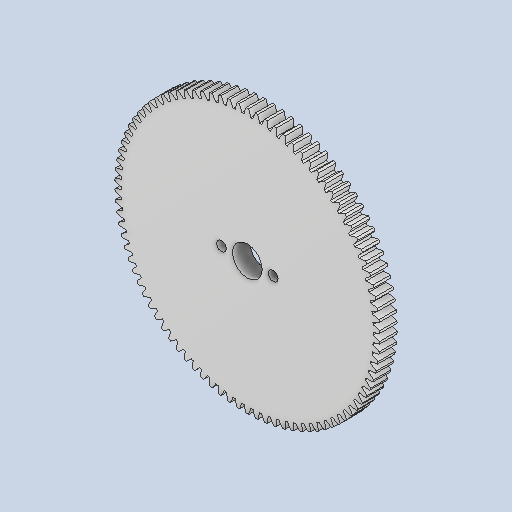
# Autodesk Inventor part: 平歯車1
Saved by Autodesk Inventor 2025.2 (Build 292293000, 293)
## iProperties
CustomPartVersion: 1
Created: 2024-12-08
Part Number: 平歯車1
Material: ABS プラスチック
Document SubType Name: Modeling
Designer: haruy
Categories: <?xml version="1.0" encoding="UTF-16"?> <MemberInstance><Categories><FamilyTemplate><FamilyTemplateParameter ValueType="xs:double" Id="1" ObjectReferenceKey="da_z" ObjectType="kUserParameterObject"/><FamilyTemplateParameter ValueType="xs:double" Id="2" ObjectReferenceKey="da_b" ObjectType="kUserParameterObject"/><FamilyTemplateParameter ValueType="xs:double" Id="3" ObjectReferenceKey="da_beta" ObjectType="kUserParameterObject"/><FamilyTemplateParameter ValueType="xs:double" Id="4" ObjectReferenceKey="da_da" ObjectType="kUserParameterObject"/><FamilyTemplateParameter ValueType="xs:double" Id="5" ObjectReferenceKey="da_aw" ObjectType="kUserParameterObject"/><FamilyTemplateParameter ValueType="xs:string" Id="6" ObjectReferenceKey="EAIAABAAAACIAQAAAAAAAIAAAAAAAAAA" ObjectType="83910656" SubObjectId="SurfaceGeometry"/></FamilyTemplate><ParamToTemplateMap><ParamToTemplate CategoryParameter="//CategoryParameter[@InternalName='046C89C9-8512-4d59-83FE-43B91F4F132A']" TemplateParameter="1"/><ParamToTemplate CategoryParameter="//CategoryParameter[@InternalName='2552DF32-E462-4b46-AEBF-C6C7768E72AC']" TemplateParameter="2"/><ParamToTemplate CategoryParameter="//CategoryParameter[@InternalName='C9EE641D-15FC-4fae-A226-E94C4372FDD7']" TemplateParameter="3"/><ParamToTemplate><ParamToTemplate CategoryParameter="//CategoryParameter[@InternalName='00B6519A-459B-49c7-AD84-2E56D39A5744']" ConstantValue="0.000000"/></ParamToTemplate><ParamToTemplate><ParamToTemplate CategoryParameter="//CategoryParameter[@InternalName='04B31F0E-C7A6-4894-AA32-9629BEFACF47']" ConstantValue="1.000000"/></ParamToTemplate><ParamToTemplate><ParamToTemplate CategoryParameter="//CategoryParameter[@InternalName='43CBEC2E-7847-49e7-A936-2F7889FCB2D9']" ConstantValue="0.250000"/></ParamToTemplate><ParamToTemplate><ParamToTemplate CategoryParameter="//CategoryParameter[@InternalName='B1EFC894-105D-4ebd-86BF-FA20ED196853']" ConstantValue="0.350000"/></ParamToTemplate><ParamToTemplate><ParamToTemplate CategoryParameter="//CategoryParameter[@InternalName='51175063-3D10-4879-93E8-6246FE8B403D']" ConstantValue="2060000000.000000"/></ParamToTemplate><ParamToTemplate><ParamToTemplate CategoryParameter="//CategoryParameter[@InternalName='A3A52E27-4454-46a9-B0BD-C932399B70AF']" ConstantValue="0.300000"/></ParamToTemplate><ParamToTemplate><ParamToTemplate CategoryParameter="//CategoryParameter[@InternalName='91B76062-C214-41d9-B1B9-14D2AB99603D']" ConstantValue="0.100000"/></ParamToTemplate><ParamToTemplate><ParamToTemplate CategoryParameter="//CategoryParameter[@InternalName='374E806E-8B8A-4dda-A9AA-1039D6500AD2']" ConstantValue="10.000000"/></ParamToTemplate><ParamToTemplate><ParamToTemplate CategoryParameter="//CategoryParameter[@InternalName='2D373A89-B862-43d6-8D0B-0CBF12AB9F6C']" ConstantValue="0.349066"/></ParamToTemplate><ParamToTemplate CategoryParameter="//CategoryParameter[@InternalName='37777632-D6A2-4fac-9D53-DB8ACD95C989']" TemplateParameter="4"/><ParamToTemplate CategoryParameter="//CategoryParameter[@InternalName='FD1017F1-B727-4f7e-9707-0F86F1FF9423']" TemplateParameter="5"/><ParamToTemplate><ParamToTemplate CategoryParameter="//CategoryParameter[@InternalName='9E1B4470-B2D3-4ff1-B813-535BB4CDF51A']" ConstantValue="3520000.000000"/></ParamToTemplate><ParamToTemplate><ParamToTemplate CategoryParameter="//CategoryParameter[@InternalName='F8452263-BFF6-458c-9FB1-07C4B99E95CD']" ConstantValue="11400000.000000"/></ParamToTemplate><ParamToTemplate><ParamToTemplate CategoryParameter="//CategoryParameter[@InternalName='3E3BB259-FD49-497f-8171-6EBC954A3479']" ConstantValue="2.000000"/></ParamToTemplate><ParamToTemplate CategoryParameter="//CategoryParameter[@InternalName='27C3BAF2-7550-4e4b-AE2C-0DB134B7D9B7']" TemplateParameter="6"/></ParamToTemplateMap><Category DisplayName="Gear" InternalName="DC85795E-93AB-48d5-8EEE-5A27447B64BD" Mnemonic="Gear"><CategoryParameter DisplayName="z" InternalName="046C89C9-8512-4d59-83FE-43B91F4F132A" Mnemonic="z"/><CategoryParameter DisplayName="b" InternalName="2552DF32-E462-4b46-AEBF-C6C7768E72AC" Mnemonic="b"/><CategoryParameter DisplayName="||b|" InternalName="C9EE641D-15FC-4fae-A226-E94C4372FDD7" Mnemonic="beta"/><CategoryParameter DisplayName="x" InternalName="00B6519A-459B-49c7-AD84-2E56D39A5744" Mnemonic="x"/><CategoryParameter DisplayName="a*" InternalName="04B31F0E-C7A6-4894-AA32-9629BEFACF47" Mnemonic="a"/><CategoryParameter DisplayName="c*" InternalName="43CBEC2E-7847-49e7-A936-2F7889FCB2D9" Mnemonic="c"/><CategoryParameter DisplayName="r|.f|*" InternalName="B1EFC894-105D-4ebd-86BF-FA20ED196853" Mnemonic="rf"/><CategoryParameter DisplayName="E" InternalName="51175063-3D10-4879-93E8-6246FE8B403D" Mnemonic="E"/><CategoryParameter DisplayName="||m|" InternalName="A3A52E27-4454-46a9-B0BD-C932399B70AF" Mnemonic="mi"/><Category DisplayName="SpurGear" InternalName="26C5A22E-A91E-4dfd-A3B3-23CCAFAE1764" Mnemonic="SpurGear"><CategoryParameter DisplayName="m" InternalName="91B76062-C214-41d9-B1B9-14D2AB99603D" Mnemonic="m"/><CategoryParameter DisplayName="P" InternalName="374E806E-8B8A-4dda-A9AA-1039D6500AD2" Mnemonic="PP"/><CategoryParameter DisplayName="||a|" InternalName="2D373A89-B862-43d6-8D0B-0CBF12AB9F6C" Mnemonic="alpha"/><CategoryParameter DisplayName="d|.a|" InternalName="37777632-D6A2-4fac-9D53-DB8ACD95C989" Mnemonic="da"/><CategoryParameter DisplayName="a|.w|" InternalName="FD1017F1-B727-4f7e-9707-0F86F1FF9423" Mnemonic="aw"/><CategoryParameter DisplayName="||s||.Flim|" InternalName="9E1B4470-B2D3-4ff1-B813-535BB4CDF51A" Mnemonic="sFlim"/><CategoryParameter DisplayName="||s||.Hlim|" InternalName="F8452263-BFF6-458c-9FB1-07C4B99E95CD" Mnemonic="sHlim"/><CategoryParameter DisplayName="タイプ" InternalName="3E3BB259-FD49-497f-8171-6EBC954A3479" Mnemonic="type"/><CategoryParameter DisplayName="PitchDiameter" InternalName="27C3BAF2-7550-4e4b-AE2C-0DB134B7D9B7" Mnemonic="IDS_PITCHDIAM"/></Category></Category></Categories></MemberInstance>
Density: 1.06 g/cm^3
Appearance: 滑らか - 白
d16: 60.000 mm
d17: 0.000 mm
d41: 0.000 mm
d43: 60.000 mm
d46: 60.000 mm
d47: 0.000 mm
d48: 0.000 mm
Author: haruy
Autodesk Inventor part; units mm, degrees
sketch "Sketch1" plane through (0, 0, 0) normal (0, 0, 1) x (1, 0, 0)
  circle A0 centre (0, 0) radius 46
  dimension "d0" = 92
  constraints: 1 centre point
  measures "d0" diameter of A0
extrude "Extrusion1" add sketch "Sketch1" along normal blind 6
ref_plane "Work Plane2" through (0, 0, 3) normal (0, 0, 1) x (1, 0, 0)
sketch "Sketch2" plane through (0, 0, 0) normal (0, 0, -1) x (-1, 0, 0)
  circle A0 centre (0, 0) radius 46 projected
  circle A1 centre (0, 0) radius 45
  dimension "d3" = 90
  constraints: 1 centre point, 1 coincident
  measures "d3" diameter of A1
surface extrude "ピッチ円直径" sketch "Sketch2" against normal through all shown no curves A1
ref_plane "Work Plane8" through (0, 0, 0) normal (0.9993908, 0.0348995, 0) x (0, 0, 1)
ref_plane "Work Plane9" through (0, 0, 0) normal (1, 0, 0) x (0, 1, 0)
spur gear teeth "平歯車" teeth 90 pitch diameter 90 tip diameter 92 root diameter 87.5 face width 6 start plane through (0, 0, 0) normal (0, 0, -1) x (-1, 0, 0)
sketch "スケッチ3" plane through (0, 0, 6) normal (0, 0, 1) x (1, 0, 0)
  circle A0 centre (0, 0) radius 5.15
  circle A1 centre (-9, 0) radius 1.7
  circle A2 centre (9, 0) radius 1.7
  dimension "d49" = 10.3
  dimension "d50" = 3.4
  dimension "d51" = 9
  dimension "d54" = 360
  constraints: 3 centre point, 1 coincident, 5 other
  measures "d49" diameter of A0
  measures "d50" diameter of A1
  measures "d51" distance of A1.centre point (0, 0)
extrude "押し出し2" cut sketch "スケッチ3" against normal blind 10
sketch "スケッチ4" plane through (0, 0, 6) normal (0, 0, 1) x (1, 0, 0)
  circle A0 centre (-9, 0) radius 1.7 projected
  circle A1 centre (9, 0) radius 1.7 projected
  circle A2 centre (0, 0) radius 5.15 projected
  arc A3 (-3.6091, 45.8582) -> (-4.1933, 43.5486) centre (9.4502, 41.3267) ccw projected
  arc A4 (-4.1933, 43.5486) -> (-4.9526, 43.4688) centre (0, 0) ccw projected
  arc A5 (-4.9526, 43.4688) -> (-6.0042, 45.6065) centre (-17.8359, 38.4588) ccw projected
  arc A6 (-6.0042, 45.6065) -> (-6.7992, 45.4947) centre (0, 0) ccw projected
  arc A7 (-6.7992, 45.4947) -> (-7.2208, 43.15) centre (6.5443, 41.8852) ccw projected
  arc A8 (-7.2208, 43.15) -> (-7.9728, 43.0174) centre (0, 0) ccw projected
  arc A9 (-7.9728, 43.0174) -> (-9.1709, 45.0765) centre (-20.4752, 37.1209) ccw projected
  arc A10 (-9.1709, 45.0765) -> (-9.9562, 44.9096) centre (0, 0) ccw projected
  arc A11 (-9.9562, 44.9096) -> (-10.2132, 42.5412) centre (3.6066, 42.2397) ccw projected
  arc A12 (-10.2132, 42.5412) -> (-10.9541, 42.3565) centre (0, 0) ccw projected
  arc A13 (-10.9541, 42.3565) -> (-12.293, 44.327) centre (-23.0148, 35.6022) ccw projected
  arc A14 (-12.293, 44.327) -> (-13.0647, 44.1057) centre (0, 0) ccw projected
  arc A15 (-13.0647, 44.1057) -> (-13.1559, 41.7251) centre (0.6514, 42.3884) ccw projected
  arc A16 (-13.1559, 41.7251) -> (-13.8821, 41.4892) centre (0, 0) ccw projected
  arc A17 (-13.8821, 41.4892) -> (-15.3551, 43.3615) centre (-25.4422, 33.91) ccw projected
  arc A18 (-15.3551, 43.3615) -> (-16.1095, 43.0869) centre (0, 0) ccw projected
  arc A19 (-16.1095, 43.0869) -> (-16.0344, 40.7058) centre (-2.3071, 42.3305) ccw projected
  arc A20 (-16.0344, 40.7058) -> (-16.7424, 40.4197) centre (0, 0) ccw projected
  arc A21 (-16.7424, 40.4197) -> (-18.3425, 42.1848) centre (-27.7457, 32.0527) ccw projected
  arc A22 (-18.3425, 42.1848) -> (-19.0759, 41.8582) centre (0, 0) ccw projected
  arc A23 (-19.0759, 41.8582) -> (-18.8349, 39.4881) centre (-5.2543, 42.0665) ccw projected
  arc A24 (-18.8349, 39.4881) -> (-19.5212, 39.1534) centre (0, 0) ccw projected
  arc A25 (-19.5212, 39.1534) -> (-21.2404, 40.8025) centre (-29.914, 30.0392) ccw projected
  arc A26 (-21.2404, 40.8025) -> (-21.9493, 40.4256) centre (0, 0) ccw projected
  arc A27 (-21.9493, 40.4256) -> (-21.5435, 38.0781) centre (-8.1759, 41.5975) ccw projected
  arc A28 (-21.5435, 38.0781) -> (-22.2048, 37.6963) centre (0, 0) ccw projected
  arc A29 (-22.2048, 37.6963) -> (-24.0349, 39.2214) centre (-31.9365, 27.8793) ccw projected
  arc A30 (-24.0349, 39.2214) -> (-24.7158, 38.796) centre (0, 0) ccw projected
  arc A31 (-24.7158, 38.796) -> (-24.1472, 36.4825) centre (-11.0577, 40.9258) ccw projected
  arc A32 (-24.1472, 36.4825) -> (-24.7803, 36.0555) centre (0, 0) ccw projected
  arc A33 (-24.7803, 36.0555) -> (-26.7123, 37.4493) centre (-33.8035, 25.5836) ccw projected
  arc A34 (-26.7123, 37.4493) -> (-27.3618, 36.9774) centre (0, 0) ccw projected
  arc A35 (-27.3618, 36.9774) -> (-26.6333, 34.7092) centre (-13.8856, 40.0548) ccw projected
  arc A36 (-26.6333, 34.7092) -> (-27.235, 34.2391) centre (0, 0) ccw projected
  arc A37 (-27.235, 34.2391) -> (-29.2596, 35.4947) centre (-35.5058, 23.1633) ccw projected
  arc A38 (-29.2596, 35.4947) -> (-29.8746, 34.9787) centre (0, 0) ccw projected
  arc A39 (-29.8746, 34.9787) -> (-28.9896, 32.7668) centre (-16.6459, 38.9886) ccw projected
  arc A40 (-28.9896, 32.7668) -> (-29.5571, 32.2559) centre (0, 0) ccw projected
  arc A41 (-29.5571, 32.2559) -> (-31.6643, 33.3672) centre (-37.0351, 20.6301) ccw projected
  arc A42 (-31.6643, 33.3672) -> (-32.2418, 32.8095) centre (0, 0) ccw projected
  arc A43 (-32.2418, 32.8095) -> (-31.2047, 30.6648) centre (-19.325, 37.7325) ccw projected
  arc A44 (-31.2047, 30.6648) -> (-31.7351, 30.1155) centre (0, 0) ccw projected
  arc A45 (-31.7351, 30.1155) -> (-33.9148, 31.0771) centre (-38.3839, 17.9964) ccw projected
  arc A46 (-33.9148, 31.0771) -> (-34.452, 30.4805) centre (0, 0) ccw projected
  arc A47 (-34.452, 30.4805) -> (-33.2678, 28.4134) centre (-21.91, 36.2925) ccw projected
  arc A48 (-33.2678, 28.4134) -> (-33.7586, 27.8284) centre (0, 0) ccw projected
  arc A49 (-33.7586, 27.8284) -> (-36, 28.6357) centre (-39.5458, 15.275) ccw projected
  arc A50 (-36, 28.6357) -> (-36.4943, 28.003) centre (0, 0) ccw projected
  arc A51 (-36.4943, 28.003) -> (-35.1687, 26.0235) centre (-24.3883, 34.6758) ccw projected
  arc A52 (-35.1687, 26.0235) -> (-35.6176, 25.4058) centre (0, 0) ccw projected
  arc A53 (-35.6176, 25.4058) -> (-37.9098, 26.0547) centre (-40.515, 12.4792) ccw projected
  arc A54 (-37.9098, 26.0547) -> (-38.3587, 25.3891) centre (0, 0) ccw projected
  arc A55 (-38.3587, 25.3891) -> (-36.8984, 23.5069) centre (-26.7477, 32.8901) ccw projected
  arc A56 (-36.8984, 23.5069) -> (-37.303, 22.8593) centre (0, 0) ccw projected
  arc A57 (-37.303, 22.8593) -> (-39.6349, 23.3468) centre (-41.2868, 9.6227) ccw projected
  arc A58 (-39.6349, 23.3468) -> (-40.0364, 22.6515) centre (0, 0) ccw projected
  arc A59 (-40.0364, 22.6515) -> (-38.4482, 20.8757) centre (-28.9769, 30.9441) ccw projected
  arc A60 (-38.4482, 20.8757) -> (-38.8067, 20.2015) centre (0, 0) ccw projected
  arc A61 (-38.8067, 20.2015) -> (-41.167, 20.5251) centre (-41.8575, 6.7192) ccw projected
  arc A62 (-41.167, 20.5251) -> (-41.5189, 19.8035) centre (0, 0) ccw projected
  arc A63 (-41.5189, 19.8035) -> (-39.8108, 18.1428) centre (-31.0648, 28.8474) ccw projected
  arc A64 (-39.8108, 18.1428) -> (-40.1214, 17.4453) centre (0, 0) ccw projected
  arc A65 (-40.1214, 17.4453) -> (-42.4985, 17.6034) centre (-42.2242, 3.783) ccw projected
  arc A66 (-42.4985, 17.6034) -> (-42.7992, 16.8591) centre (0, 0) ccw projected
  arc A67 (-42.7992, 16.8591) -> (-40.9794, 15.3216) centre (-33.0015, 26.6102) ccw projected
  arc A68 (-40.9794, 15.3216) -> (-41.2406, 14.6041) centre (0, 0) ccw projected
  arc A69 (-41.2406, 14.6041) -> (-43.6229, 14.596) centre (-42.3853, 0.8284) ccw projected
  arc A70 (-43.6229, 14.596) -> (-43.871, 13.8325) centre (0, 0) ccw projected
  arc A71 (-43.871, 13.8325) -> (-41.9484, 12.4257) centre (-34.7773, 24.2433) ccw projected
  arc A72 (-41.9484, 12.4257) -> (-42.1588, 11.6917) centre (0, 0) ccw projected
  arc A73 (-42.1588, 11.6917) -> (-44.5348, 11.5175) centre (-42.3398, -2.1303) ccw projected
  arc A74 (-44.5348, 11.5175) -> (-44.729, 10.7385) centre (0, 0) ccw projected
  arc A75 (-44.729, 10.7385) -> (-42.713, 9.4692) centre (-36.3837, 21.7583) ccw projected
  arc A76 (-42.713, 9.4692) -> (-42.8717, 8.7223) centre (0, 0) ccw projected
  arc A77 (-42.8717, 8.7223) -> (-45.2297, 8.3828) centre (-42.0881, -5.0786) ccw projected
  arc A78 (-45.2297, 8.3828) -> (-45.3691, 7.5922) centre (0, 0) ccw projected
  arc A79 (-45.3691, 7.5922) -> (-43.2694, 6.4667) centre (-37.8129, 19.1673) ccw projected
  arc A80 (-43.2694, 6.4667) -> (-43.3757, 5.7105) centre (0, 0) ccw projected
  arc A81 (-43.3757, 5.7105) -> (-45.7043, 5.2073) centre (-41.6313, -8.0021) ccw projected
  arc A82 (-45.7043, 5.2073) -> (-45.7882, 4.4089) centre (0, 0) ccw projected
  arc A83 (-45.7882, 4.4089) -> (-43.6151, 3.4326) centre (-39.0578, 16.4829) ccw projected
  arc A84 (-43.6151, 3.4326) -> (-43.6684, 2.6709) centre (0, 0) ccw projected
  arc A85 (-43.6684, 2.6709) -> (-45.9562, 2.0065) centre (-40.9717, -10.8867) ccw projected
  arc A86 (-45.9562, 2.0065) -> (-45.9842, 1.2041) centre (0, 0) ccw projected
  arc A87 (-45.9842, 1.2041) -> (-43.7483, 0.3818) centre (-40.1124, 13.7182) ccw projected
  arc A88 (-43.7483, 0.3818) -> (-43.7483, -0.3818) centre (0, 0) ccw projected
  arc A89 (-43.7483, -0.3818) -> (-45.9842, -1.2041) centre (-40.1124, -13.7182) ccw projected
  arc A90 (-45.9842, -1.2041) -> (-45.9562, -2.0065) centre (0, 0) ccw projected
  arc A91 (-45.9562, -2.0065) -> (-43.6684, -2.6709) centre (-40.9717, 10.8867) ccw projected
  arc A92 (-43.6684, -2.6709) -> (-43.6151, -3.4326) centre (0, 0) ccw projected
  arc A93 (-43.6151, -3.4326) -> (-45.7882, -4.4089) centre (-39.0578, -16.4829) ccw projected
  arc A94 (-45.7882, -4.4089) -> (-45.7043, -5.2073) centre (0, 0) ccw projected
  arc A95 (-45.7043, -5.2073) -> (-43.3757, -5.7105) centre (-41.6313, 8.0021) ccw projected
  arc A96 (-43.3757, -5.7105) -> (-43.2694, -6.4667) centre (0, 0) ccw projected
  arc A97 (-43.2694, -6.4667) -> (-45.3691, -7.5922) centre (-37.8129, -19.1673) ccw projected
  arc A98 (-45.3691, -7.5922) -> (-45.2297, -8.3828) centre (0, 0) ccw projected
  arc A99 (-45.2297, -8.3828) -> (-42.8717, -8.7223) centre (-42.0881, 5.0786) ccw projected
  arc A100 (-42.8717, -8.7223) -> (-42.713, -9.4692) centre (0, 0) ccw projected
  arc A101 (-42.713, -9.4692) -> (-44.729, -10.7385) centre (-36.3837, -21.7583) ccw projected
  arc A102 (-44.729, -10.7385) -> (-44.5348, -11.5175) centre (0, 0) ccw projected
  arc A103 (-44.5348, -11.5175) -> (-42.1588, -11.6917) centre (-42.3398, 2.1303) ccw projected
  arc A104 (-42.1588, -11.6917) -> (-41.9484, -12.4257) centre (0, 0) ccw projected
  arc A105 (-41.9484, -12.4257) -> (-43.871, -13.8325) centre (-34.7773, -24.2433) ccw projected
  arc A106 (-43.871, -13.8325) -> (-43.6229, -14.596) centre (0, 0) ccw projected
  arc A107 (-43.6229, -14.596) -> (-41.2406, -14.6041) centre (-42.3853, -0.8284) ccw projected
  arc A108 (-41.2406, -14.6041) -> (-40.9794, -15.3216) centre (0, 0) ccw projected
  arc A109 (-40.9794, -15.3216) -> (-42.7992, -16.8591) centre (-33.0015, -26.6102) ccw projected
  arc A110 (-42.7992, -16.8591) -> (-42.4985, -17.6034) centre (0, 0) ccw projected
  arc A111 (-42.4985, -17.6034) -> (-40.1214, -17.4453) centre (-42.2242, -3.783) ccw projected
  arc A112 (-40.1214, -17.4453) -> (-39.8108, -18.1428) centre (0, 0) ccw projected
  arc A113 (-39.8108, -18.1428) -> (-41.5189, -19.8035) centre (-31.0648, -28.8474) ccw projected
  arc A114 (-41.5189, -19.8035) -> (-41.167, -20.5251) centre (0, 0) ccw projected
  arc A115 (-41.167, -20.5251) -> (-38.8067, -20.2015) centre (-41.8575, -6.7192) ccw projected
  arc A116 (-38.8067, -20.2015) -> (-38.4482, -20.8757) centre (0, 0) ccw projected
  arc A117 (-38.4482, -20.8757) -> (-40.0364, -22.6515) centre (-28.9769, -30.9441) ccw projected
  arc A118 (-40.0364, -22.6515) -> (-39.6349, -23.3468) centre (0, 0) ccw projected
  arc A119 (-39.6349, -23.3468) -> (-37.303, -22.8593) centre (-41.2868, -9.6227) ccw projected
  arc A120 (-37.303, -22.8593) -> (-36.8984, -23.5069) centre (0, 0) ccw projected
  arc A121 (-36.8984, -23.5069) -> (-38.3587, -25.3891) centre (-26.7477, -32.8901) ccw projected
  arc A122 (-38.3587, -25.3891) -> (-37.9098, -26.0547) centre (0, 0) ccw projected
  arc A123 (-37.9098, -26.0547) -> (-35.6176, -25.4058) centre (-40.515, -12.4792) ccw projected
  arc A124 (-35.6176, -25.4058) -> (-35.1687, -26.0235) centre (0, 0) ccw projected
  arc A125 (-35.1687, -26.0235) -> (-36.4943, -28.003) centre (-24.3883, -34.6758) ccw projected
  arc A126 (-36.4943, -28.003) -> (-36, -28.6357) centre (0, 0) ccw projected
  arc A127 (-36, -28.6357) -> (-33.7586, -27.8284) centre (-39.5458, -15.275) ccw projected
  arc A128 (-33.7586, -27.8284) -> (-33.2678, -28.4134) centre (0, 0) ccw projected
  arc A129 (-33.2678, -28.4134) -> (-34.452, -30.4805) centre (-21.91, -36.2925) ccw projected
  arc A130 (-34.452, -30.4805) -> (-33.9148, -31.0771) centre (0, 0) ccw projected
  arc A131 (-33.9148, -31.0771) -> (-31.7351, -30.1155) centre (-38.3839, -17.9964) ccw projected
  arc A132 (-31.7351, -30.1155) -> (-31.2047, -30.6648) centre (0, 0) ccw projected
  arc A133 (-31.2047, -30.6648) -> (-32.2418, -32.8095) centre (-19.325, -37.7325) ccw projected
  arc A134 (-32.2418, -32.8095) -> (-31.6643, -33.3672) centre (0, 0) ccw projected
  arc A135 (-31.6643, -33.3672) -> (-29.5571, -32.2559) centre (-37.0351, -20.6301) ccw projected
  arc A136 (-29.5571, -32.2559) -> (-28.9896, -32.7668) centre (0, 0) ccw projected
  arc A137 (-28.9896, -32.7668) -> (-29.8746, -34.9787) centre (-16.6459, -38.9886) ccw projected
  arc A138 (-29.8746, -34.9787) -> (-29.2596, -35.4947) centre (0, 0) ccw projected
  arc A139 (-29.2596, -35.4947) -> (-27.235, -34.2391) centre (-35.5058, -23.1633) ccw projected
  arc A140 (-27.235, -34.2391) -> (-26.6333, -34.7092) centre (0, 0) ccw projected
  arc A141 (-26.6333, -34.7092) -> (-27.3618, -36.9774) centre (-13.8856, -40.0548) ccw projected
  arc A142 (-27.3618, -36.9774) -> (-26.7123, -37.4493) centre (0, 0) ccw projected
  arc A143 (-26.7123, -37.4493) -> (-24.7803, -36.0555) centre (-33.8035, -25.5836) ccw projected
  arc A144 (-24.7803, -36.0555) -> (-24.1472, -36.4825) centre (0, 0) ccw projected
  arc A145 (-24.1472, -36.4825) -> (-24.7158, -38.796) centre (-11.0577, -40.9258) ccw projected
  arc A146 (-24.7158, -38.796) -> (-24.0349, -39.2214) centre (0, 0) ccw projected
  arc A147 (-24.0349, -39.2214) -> (-22.2048, -37.6963) centre (-31.9365, -27.8793) ccw projected
  arc A148 (-22.2048, -37.6963) -> (-21.5435, -38.0781) centre (0, 0) ccw projected
  arc A149 (-21.5435, -38.0781) -> (-21.9493, -40.4256) centre (-8.1759, -41.5975) ccw projected
  arc A150 (-21.9493, -40.4256) -> (-21.2404, -40.8025) centre (0, 0) ccw projected
  arc A151 (-21.2404, -40.8025) -> (-19.5212, -39.1534) centre (-29.914, -30.0392) ccw projected
  arc A152 (-19.5212, -39.1534) -> (-18.8349, -39.4881) centre (0, 0) ccw projected
  arc A153 (-18.8349, -39.4881) -> (-19.0759, -41.8582) centre (-5.2543, -42.0665) ccw projected
  arc A154 (-19.0759, -41.8582) -> (-18.3425, -42.1848) centre (0, 0) ccw projected
  arc A155 (-18.3425, -42.1848) -> (-16.7424, -40.4197) centre (-27.7457, -32.0527) ccw projected
  arc A156 (-16.7424, -40.4197) -> (-16.0344, -40.7058) centre (0, 0) ccw projected
  arc A157 (-16.0344, -40.7058) -> (-16.1095, -43.0869) centre (-2.3071, -42.3305) ccw projected
  arc A158 (-16.1095, -43.0869) -> (-15.3551, -43.3615) centre (0, 0) ccw projected
  arc A159 (-15.3551, -43.3615) -> (-13.8821, -41.4892) centre (-25.4422, -33.91) ccw projected
  arc A160 (-13.8821, -41.4892) -> (-13.1559, -41.7251) centre (0, 0) ccw projected
  arc A161 (-13.1559, -41.7251) -> (-13.0647, -44.1057) centre (0.6514, -42.3884) ccw projected
  arc A162 (-13.0647, -44.1057) -> (-12.293, -44.327) centre (0, 0) ccw projected
  arc A163 (-12.293, -44.327) -> (-10.9541, -42.3565) centre (-23.0148, -35.6022) ccw projected
  arc A164 (-10.9541, -42.3565) -> (-10.2132, -42.5412) centre (0, 0) ccw projected
  arc A165 (-10.2132, -42.5412) -> (-9.9562, -44.9096) centre (3.6066, -42.2397) ccw projected
  arc A166 (-9.9562, -44.9096) -> (-9.1709, -45.0765) centre (0, 0) ccw projected
  arc A167 (-9.1709, -45.0765) -> (-7.9728, -43.0174) centre (-20.4752, -37.1209) ccw projected
  arc A168 (-7.9728, -43.0174) -> (-7.2208, -43.15) centre (0, 0) ccw projected
  arc A169 (-7.2208, -43.15) -> (-6.7992, -45.4947) centre (6.5443, -41.8852) ccw projected
  arc A170 (-6.7992, -45.4947) -> (-6.0042, -45.6065) centre (0, 0) ccw projected
  arc A171 (-6.0042, -45.6065) -> (-4.9526, -43.4688) centre (-17.8359, -38.4588) ccw projected
  arc A172 (-4.9526, -43.4688) -> (-4.1933, -43.5486) centre (0, 0) ccw projected
  arc A173 (-4.1933, -43.5486) -> (-3.6091, -45.8582) centre (9.4502, -41.3267) ccw projected
  arc A174 (-3.6091, -45.8582) -> (-2.8082, -45.9142) centre (0, 0) ccw projected
  arc A175 (-2.8082, -45.9142) -> (-1.9083, -43.7084) centre (-15.1097, -39.6093) ccw projected
  arc A176 (-1.9083, -43.7084) -> (-1.1452, -43.735) centre (0, 0) ccw projected
  arc A177 (-1.1452, -43.735) -> (-0.4014, -45.9982) centre (12.3099, -40.5668) ccw projected
  arc A178 (-0.4014, -45.9982) -> (0.4014, -45.9982) centre (0, 0) ccw projected
  arc A179 (0.4014, -45.9982) -> (1.1452, -43.735) centre (-12.3099, -40.5668) ccw projected
  arc A180 (1.1452, -43.735) -> (1.9083, -43.7084) centre (0, 0) ccw projected
  arc A181 (1.9083, -43.7084) -> (2.8082, -45.9142) centre (15.1097, -39.6093) ccw projected
  arc A182 (2.8082, -45.9142) -> (3.6091, -45.8582) centre (0, 0) ccw projected
  arc A183 (3.6091, -45.8582) -> (4.1933, -43.5486) centre (-9.4502, -41.3267) ccw projected
  arc A184 (4.1933, -43.5486) -> (4.9526, -43.4688) centre (0, 0) ccw projected
  arc A185 (4.9526, -43.4688) -> (6.0042, -45.6065) centre (17.8359, -38.4588) ccw projected
  arc A186 (6.0042, -45.6065) -> (6.7992, -45.4947) centre (0, 0) ccw projected
  arc A187 (6.7992, -45.4947) -> (7.2208, -43.15) centre (-6.5443, -41.8852) ccw projected
  arc A188 (7.2208, -43.15) -> (7.9728, -43.0174) centre (0, 0) ccw projected
  arc A189 (7.9728, -43.0174) -> (9.1709, -45.0765) centre (20.4752, -37.1209) ccw projected
  arc A190 (9.1709, -45.0765) -> (9.9562, -44.9096) centre (0, 0) ccw projected
  arc A191 (9.9562, -44.9096) -> (10.2132, -42.5412) centre (-3.6066, -42.2397) ccw projected
  arc A192 (10.2132, -42.5412) -> (10.9541, -42.3565) centre (0, 0) ccw projected
  arc A193 (10.9541, -42.3565) -> (12.293, -44.327) centre (23.0148, -35.6022) ccw projected
  arc A194 (12.293, -44.327) -> (13.0647, -44.1057) centre (0, 0) ccw projected
  arc A195 (13.0647, -44.1057) -> (13.1559, -41.7251) centre (-0.6514, -42.3884) ccw projected
  arc A196 (13.1559, -41.7251) -> (13.8821, -41.4892) centre (0, 0) ccw projected
  arc A197 (13.8821, -41.4892) -> (15.3551, -43.3615) centre (25.4422, -33.91) ccw projected
  arc A198 (15.3551, -43.3615) -> (16.1095, -43.0869) centre (0, 0) ccw projected
  arc A199 (16.1095, -43.0869) -> (16.0344, -40.7058) centre (2.3071, -42.3305) ccw projected
  arc A200 (16.0344, -40.7058) -> (16.7424, -40.4197) centre (0, 0) ccw projected
  arc A201 (16.7424, -40.4197) -> (18.3425, -42.1848) centre (27.7457, -32.0527) ccw projected
  arc A202 (18.3425, -42.1848) -> (19.0759, -41.8582) centre (0, 0) ccw projected
  arc A203 (19.0759, -41.8582) -> (18.8349, -39.4881) centre (5.2543, -42.0665) ccw projected
  arc A204 (18.8349, -39.4881) -> (19.5212, -39.1534) centre (0, 0) ccw projected
  arc A205 (19.5212, -39.1534) -> (21.2404, -40.8025) centre (29.914, -30.0392) ccw projected
  arc A206 (21.2404, -40.8025) -> (21.9493, -40.4256) centre (0, 0) ccw projected
  arc A207 (21.9493, -40.4256) -> (21.5435, -38.0781) centre (8.1759, -41.5975) ccw projected
  arc A208 (21.5435, -38.0781) -> (22.2048, -37.6963) centre (0, 0) ccw projected
  arc A209 (22.2048, -37.6963) -> (24.0349, -39.2214) centre (31.9365, -27.8793) ccw projected
  arc A210 (24.0349, -39.2214) -> (24.7158, -38.796) centre (0, 0) ccw projected
  arc A211 (24.7158, -38.796) -> (24.1472, -36.4825) centre (11.0577, -40.9258) ccw projected
  arc A212 (24.1472, -36.4825) -> (24.7803, -36.0555) centre (0, 0) ccw projected
  arc A213 (24.7803, -36.0555) -> (26.7123, -37.4493) centre (33.8035, -25.5836) ccw projected
  arc A214 (26.7123, -37.4493) -> (27.3618, -36.9774) centre (0, 0) ccw projected
  arc A215 (27.3618, -36.9774) -> (26.6333, -34.7092) centre (13.8856, -40.0548) ccw projected
  arc A216 (26.6333, -34.7092) -> (27.235, -34.2391) centre (0, 0) ccw projected
  arc A217 (27.235, -34.2391) -> (29.2596, -35.4947) centre (35.5058, -23.1633) ccw projected
  arc A218 (29.2596, -35.4947) -> (29.8746, -34.9787) centre (0, 0) ccw projected
  arc A219 (29.8746, -34.9787) -> (28.9896, -32.7668) centre (16.6459, -38.9886) ccw projected
  arc A220 (28.9896, -32.7668) -> (29.5571, -32.2559) centre (0, 0) ccw projected
  arc A221 (29.5571, -32.2559) -> (31.6643, -33.3672) centre (37.0351, -20.6301) ccw projected
  arc A222 (31.6643, -33.3672) -> (32.2418, -32.8095) centre (0, 0) ccw projected
  arc A223 (32.2418, -32.8095) -> (31.2047, -30.6648) centre (19.325, -37.7325) ccw projected
  arc A224 (31.2047, -30.6648) -> (31.7351, -30.1155) centre (0, 0) ccw projected
  arc A225 (31.7351, -30.1155) -> (33.9148, -31.0771) centre (38.3839, -17.9964) ccw projected
  arc A226 (33.9148, -31.0771) -> (34.452, -30.4805) centre (0, 0) ccw projected
  arc A227 (34.452, -30.4805) -> (33.2678, -28.4134) centre (21.91, -36.2925) ccw projected
  arc A228 (33.2678, -28.4134) -> (33.7586, -27.8284) centre (0, 0) ccw projected
  arc A229 (33.7586, -27.8284) -> (36, -28.6357) centre (39.5458, -15.275) ccw projected
  arc A230 (36, -28.6357) -> (36.4943, -28.003) centre (0, 0) ccw projected
  arc A231 (36.4943, -28.003) -> (35.1687, -26.0235) centre (24.3883, -34.6758) ccw projected
  arc A232 (35.1687, -26.0235) -> (35.6176, -25.4058) centre (0, 0) ccw projected
  arc A233 (35.6176, -25.4058) -> (37.9098, -26.0547) centre (40.515, -12.4792) ccw projected
  arc A234 (37.9098, -26.0547) -> (38.3587, -25.3891) centre (0, 0) ccw projected
  arc A235 (38.3587, -25.3891) -> (36.8984, -23.5069) centre (26.7477, -32.8901) ccw projected
  arc A236 (36.8984, -23.5069) -> (37.303, -22.8593) centre (0, 0) ccw projected
  arc A237 (37.303, -22.8593) -> (39.6349, -23.3468) centre (41.2868, -9.6227) ccw projected
  arc A238 (39.6349, -23.3468) -> (40.0364, -22.6515) centre (0, 0) ccw projected
  arc A239 (40.0364, -22.6515) -> (38.4482, -20.8757) centre (28.9769, -30.9441) ccw projected
  arc A240 (38.4482, -20.8757) -> (38.8067, -20.2015) centre (0, 0) ccw projected
  arc A241 (38.8067, -20.2015) -> (41.167, -20.5251) centre (41.8575, -6.7192) ccw projected
  arc A242 (41.167, -20.5251) -> (41.5189, -19.8035) centre (0, 0) ccw projected
  arc A243 (41.5189, -19.8035) -> (39.8108, -18.1428) centre (31.0648, -28.8474) ccw projected
  arc A244 (39.8108, -18.1428) -> (40.1214, -17.4453) centre (0, 0) ccw projected
  arc A245 (40.1214, -17.4453) -> (42.4985, -17.6034) centre (42.2242, -3.783) ccw projected
  arc A246 (42.4985, -17.6034) -> (42.7992, -16.8591) centre (0, 0) ccw projected
  arc A247 (42.7992, -16.8591) -> (40.9794, -15.3216) centre (33.0015, -26.6102) ccw projected
  arc A248 (40.9794, -15.3216) -> (41.2406, -14.6041) centre (0, 0) ccw projected
  arc A249 (41.2406, -14.6041) -> (43.6229, -14.596) centre (42.3853, -0.8284) ccw projected
  arc A250 (43.6229, -14.596) -> (43.871, -13.8325) centre (0, 0) ccw projected
  arc A251 (43.871, -13.8325) -> (41.9484, -12.4257) centre (34.7773, -24.2433) ccw projected
  arc A252 (41.9484, -12.4257) -> (42.1588, -11.6917) centre (0, 0) ccw projected
  arc A253 (42.1588, -11.6917) -> (44.5348, -11.5175) centre (42.3398, 2.1303) ccw projected
  arc A254 (44.5348, -11.5175) -> (44.729, -10.7385) centre (0, 0) ccw projected
  arc A255 (44.729, -10.7385) -> (42.713, -9.4692) centre (36.3837, -21.7583) ccw projected
  arc A256 (42.713, -9.4692) -> (42.8717, -8.7223) centre (0, 0) ccw projected
  arc A257 (42.8717, -8.7223) -> (45.2297, -8.3828) centre (42.0881, 5.0786) ccw projected
  arc A258 (45.2297, -8.3828) -> (45.3691, -7.5922) centre (0, 0) ccw projected
  arc A259 (45.3691, -7.5922) -> (43.2694, -6.4667) centre (37.8129, -19.1673) ccw projected
  arc A260 (43.2694, -6.4667) -> (43.3757, -5.7105) centre (0, 0) ccw projected
  arc A261 (43.3757, -5.7105) -> (45.7043, -5.2073) centre (41.6313, 8.0021) ccw projected
  arc A262 (45.7043, -5.2073) -> (45.7882, -4.4089) centre (0, 0) ccw projected
  arc A263 (45.7882, -4.4089) -> (43.6151, -3.4326) centre (39.0578, -16.4829) ccw projected
  arc A264 (43.6151, -3.4326) -> (43.6684, -2.6709) centre (0, 0) ccw projected
  arc A265 (43.6684, -2.6709) -> (45.9562, -2.0065) centre (40.9717, 10.8867) ccw projected
  arc A266 (45.9562, -2.0065) -> (45.9842, -1.2041) centre (0, 0) ccw projected
  arc A267 (45.9842, -1.2041) -> (43.7483, -0.3818) centre (40.1124, -13.7182) ccw projected
  arc A268 (43.7483, -0.3818) -> (43.7483, 0.3818) centre (0, 0) ccw projected
  arc A269 (43.7483, 0.3818) -> (45.9842, 1.2041) centre (40.1124, 13.7182) ccw projected
  arc A270 (45.9842, 1.2041) -> (45.9562, 2.0065) centre (0, 0) ccw projected
  arc A271 (45.9562, 2.0065) -> (43.6684, 2.6709) centre (40.9717, -10.8867) ccw projected
  arc A272 (43.6684, 2.6709) -> (43.6151, 3.4326) centre (0, 0) ccw projected
  arc A273 (43.6151, 3.4326) -> (45.7882, 4.4089) centre (39.0578, 16.4829) ccw projected
  arc A274 (45.7882, 4.4089) -> (45.7043, 5.2073) centre (0, 0) ccw projected
  arc A275 (45.7043, 5.2073) -> (43.3757, 5.7105) centre (41.6313, -8.0021) ccw projected
  arc A276 (43.3757, 5.7105) -> (43.2694, 6.4667) centre (0, 0) ccw projected
  arc A277 (43.2694, 6.4667) -> (45.3691, 7.5922) centre (37.8129, 19.1673) ccw projected
  arc A278 (45.3691, 7.5922) -> (45.2297, 8.3828) centre (0, 0) ccw projected
  arc A279 (45.2297, 8.3828) -> (42.8717, 8.7223) centre (42.0881, -5.0786) ccw projected
  arc A280 (42.8717, 8.7223) -> (42.713, 9.4692) centre (0, 0) ccw projected
  arc A281 (42.713, 9.4692) -> (44.729, 10.7385) centre (36.3837, 21.7583) ccw projected
  arc A282 (44.729, 10.7385) -> (44.5348, 11.5175) centre (0, 0) ccw projected
  arc A283 (44.5348, 11.5175) -> (42.1588, 11.6917) centre (42.3398, -2.1303) ccw projected
  arc A284 (42.1588, 11.6917) -> (41.9484, 12.4257) centre (0, 0) ccw projected
  arc A285 (41.9484, 12.4257) -> (43.871, 13.8325) centre (34.7773, 24.2433) ccw projected
  arc A286 (43.871, 13.8325) -> (43.6229, 14.596) centre (0, 0) ccw projected
  arc A287 (43.6229, 14.596) -> (41.2406, 14.6041) centre (42.3853, 0.8284) ccw projected
  arc A288 (41.2406, 14.6041) -> (40.9794, 15.3216) centre (0, 0) ccw projected
  arc A289 (40.9794, 15.3216) -> (42.7992, 16.8591) centre (33.0015, 26.6102) ccw projected
  arc A290 (42.7992, 16.8591) -> (42.4985, 17.6034) centre (0, 0) ccw projected
  arc A291 (42.4985, 17.6034) -> (40.1214, 17.4453) centre (42.2242, 3.783) ccw projected
  arc A292 (40.1214, 17.4453) -> (39.8108, 18.1428) centre (0, 0) ccw projected
  arc A293 (39.8108, 18.1428) -> (41.5189, 19.8035) centre (31.0648, 28.8474) ccw projected
  arc A294 (41.5189, 19.8035) -> (41.167, 20.5251) centre (0, 0) ccw projected
  arc A295 (41.167, 20.5251) -> (38.8067, 20.2015) centre (41.8575, 6.7192) ccw projected
  arc A296 (38.8067, 20.2015) -> (38.4482, 20.8757) centre (0, 0) ccw projected
  arc A297 (38.4482, 20.8757) -> (40.0364, 22.6515) centre (28.9769, 30.9441) ccw projected
  arc A298 (40.0364, 22.6515) -> (39.6349, 23.3468) centre (0, 0) ccw projected
  arc A299 (39.6349, 23.3468) -> (37.303, 22.8593) centre (41.2868, 9.6227) ccw projected
  arc A300 (37.303, 22.8593) -> (36.8984, 23.5069) centre (0, 0) ccw projected
  arc A301 (36.8984, 23.5069) -> (38.3587, 25.3891) centre (26.7477, 32.8901) ccw projected
  arc A302 (38.3587, 25.3891) -> (37.9098, 26.0547) centre (0, 0) ccw projected
  arc A303 (37.9098, 26.0547) -> (35.6176, 25.4058) centre (40.515, 12.4792) ccw projected
  arc A304 (35.6176, 25.4058) -> (35.1687, 26.0235) centre (0, 0) ccw projected
  arc A305 (35.1687, 26.0235) -> (36.4943, 28.003) centre (24.3883, 34.6758) ccw projected
  arc A306 (36.4943, 28.003) -> (36, 28.6357) centre (0, 0) ccw projected
  arc A307 (36, 28.6357) -> (33.7586, 27.8284) centre (39.5458, 15.275) ccw projected
  arc A308 (33.7586, 27.8284) -> (33.2678, 28.4134) centre (0, 0) ccw projected
  arc A309 (33.2678, 28.4134) -> (34.452, 30.4805) centre (21.91, 36.2925) ccw projected
  arc A310 (34.452, 30.4805) -> (33.9148, 31.0771) centre (0, 0) ccw projected
  arc A311 (33.9148, 31.0771) -> (31.7351, 30.1155) centre (38.3839, 17.9964) ccw projected
  arc A312 (31.7351, 30.1155) -> (31.2047, 30.6648) centre (0, 0) ccw projected
  arc A313 (31.2047, 30.6648) -> (32.2418, 32.8095) centre (19.325, 37.7325) ccw projected
  arc A314 (32.2418, 32.8095) -> (31.6643, 33.3672) centre (0, 0) ccw projected
  arc A315 (31.6643, 33.3672) -> (29.5571, 32.2559) centre (37.0351, 20.6301) ccw projected
  arc A316 (29.5571, 32.2559) -> (28.9896, 32.7668) centre (0, 0) ccw projected
  arc A317 (28.9896, 32.7668) -> (29.8746, 34.9787) centre (16.6459, 38.9886) ccw projected
  arc A318 (29.8746, 34.9787) -> (29.2596, 35.4947) centre (0, 0) ccw projected
  arc A319 (29.2596, 35.4947) -> (27.235, 34.2391) centre (35.5058, 23.1633) ccw projected
  arc A320 (27.235, 34.2391) -> (26.6333, 34.7092) centre (0, 0) ccw projected
  arc A321 (26.6333, 34.7092) -> (27.3618, 36.9774) centre (13.8856, 40.0548) ccw projected
  arc A322 (27.3618, 36.9774) -> (26.7123, 37.4493) centre (0, 0) ccw projected
  arc A323 (26.7123, 37.4493) -> (24.7803, 36.0555) centre (33.8035, 25.5836) ccw projected
  arc A324 (24.7803, 36.0555) -> (24.1472, 36.4825) centre (0, 0) ccw projected
  arc A325 (24.1472, 36.4825) -> (24.7158, 38.796) centre (11.0577, 40.9258) ccw projected
  arc A326 (24.7158, 38.796) -> (24.0349, 39.2214) centre (0, 0) ccw projected
  arc A327 (24.0349, 39.2214) -> (22.2048, 37.6963) centre (31.9365, 27.8793) ccw projected
  arc A328 (22.2048, 37.6963) -> (21.5435, 38.0781) centre (0, 0) ccw projected
  arc A329 (21.5435, 38.0781) -> (21.9493, 40.4256) centre (8.1759, 41.5975) ccw projected
  arc A330 (21.9493, 40.4256) -> (21.2404, 40.8025) centre (0, 0) ccw projected
  arc A331 (21.2404, 40.8025) -> (19.5212, 39.1534) centre (29.914, 30.0392) ccw projected
  arc A332 (19.5212, 39.1534) -> (18.8349, 39.4881) centre (0, 0) ccw projected
  arc A333 (18.8349, 39.4881) -> (19.0759, 41.8582) centre (5.2543, 42.0665) ccw projected
  arc A334 (19.0759, 41.8582) -> (18.3425, 42.1848) centre (0, 0) ccw projected
  arc A335 (18.3425, 42.1848) -> (16.7424, 40.4197) centre (27.7457, 32.0527) ccw projected
  arc A336 (16.7424, 40.4197) -> (16.0344, 40.7058) centre (0, 0) ccw projected
  arc A337 (16.0344, 40.7058) -> (16.1095, 43.0869) centre (2.3071, 42.3305) ccw projected
  arc A338 (16.1095, 43.0869) -> (15.3551, 43.3615) centre (0, 0) ccw projected
  arc A339 (15.3551, 43.3615) -> (13.8821, 41.4892) centre (25.4422, 33.91) ccw projected
  arc A340 (13.8821, 41.4892) -> (13.1559, 41.7251) centre (0, 0) ccw projected
  arc A341 (13.1559, 41.7251) -> (13.0647, 44.1057) centre (-0.6514, 42.3884) ccw projected
  arc A342 (13.0647, 44.1057) -> (12.293, 44.327) centre (0, 0) ccw projected
  arc A343 (12.293, 44.327) -> (10.9541, 42.3565) centre (23.0148, 35.6022) ccw projected
  arc A344 (10.9541, 42.3565) -> (10.2132, 42.5412) centre (0, 0) ccw projected
  arc A345 (10.2132, 42.5412) -> (9.9562, 44.9096) centre (-3.6066, 42.2397) ccw projected
  arc A346 (9.9562, 44.9096) -> (9.1709, 45.0765) centre (0, 0) ccw projected
  arc A347 (9.1709, 45.0765) -> (7.9728, 43.0174) centre (20.4752, 37.1209) ccw projected
  arc A348 (7.9728, 43.0174) -> (7.2208, 43.15) centre (0, 0) ccw projected
  arc A349 (7.2208, 43.15) -> (6.7992, 45.4947) centre (-6.5443, 41.8852) ccw projected
  arc A350 (6.7992, 45.4947) -> (6.0042, 45.6065) centre (0, 0) ccw projected
  arc A351 (6.0042, 45.6065) -> (4.9526, 43.4688) centre (17.8359, 38.4588) ccw projected
  arc A352 (4.9526, 43.4688) -> (4.1933, 43.5486) centre (0, 0) ccw projected
  arc A353 (4.1933, 43.5486) -> (3.6091, 45.8582) centre (-9.4502, 41.3267) ccw projected
  arc A354 (3.6091, 45.8582) -> (2.8082, 45.9142) centre (0, 0) ccw projected
  arc A355 (2.8082, 45.9142) -> (1.9083, 43.7084) centre (15.1097, 39.6093) ccw projected
  arc A356 (1.9083, 43.7084) -> (1.1452, 43.735) centre (0, 0) ccw projected
  arc A357 (1.1452, 43.735) -> (0.4014, 45.9982) centre (-12.3099, 40.5668) ccw projected
  arc A358 (0.4014, 45.9982) -> (-0.4014, 45.9982) centre (0, 0) ccw projected
  arc A359 (-0.4014, 45.9982) -> (-1.1452, 43.735) centre (12.3099, 40.5668) ccw projected
  arc A360 (-1.1452, 43.735) -> (-1.9083, 43.7084) centre (0, 0) ccw projected
  arc A361 (-1.9083, 43.7084) -> (-2.8082, 45.9142) centre (-15.1097, 39.6093) ccw projected
  arc A362 (-2.8082, 45.9142) -> (-3.6091, 45.8582) centre (0, 0) ccw projected
equation "\"d0\" = da_da"
equation "\"d1\" = da_b"
equation "\"d3\" = da_d"
equation "\"d16\" = da_aw"
equation "\"d43\" = da_aw"
equation "\"d46\" = da_aw"
equation "\"da_da\" = 92"
equation "\"da_b\" = 6"
equation "\"da_d\" = 90"
equation "\"da_aw\" = 60"
body "Solid1"
body "Srf1"
